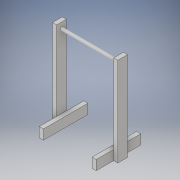
# Autodesk Inventor part: Perch
Saved by Autodesk Inventor 2017 (Build 210142000, 142)
## iProperties
Created: 2017-04-14
Part Number: Perch
Material: Generic
Document SubType Name: Modeling
Designer: Alex Tacescu
Density: 1 g/cm^3
Appearance: Default
Author: Alex Tacescu
Autodesk Inventor part; units mm, degrees
ref_plane "YZ Plane" through (0, 0, 0) normal (1, 0, 0) x (0, 1, 0)
ref_plane "XZ Plane" through (0, 0, 0) normal (0, 1, 0) x (-1, 0, 0)
ref_plane "XY Plane" through (0, 0, 0) normal (0, 0, 1) x (1, 0, 0)
sketch "Sketch1" plane through (0, 0, 0) normal (0, 1, 0) x (-1, 0, 0)
  line L0 (0, -284.48) -> (0, 284.48) projected
  line L1 (-364.49, 0) -> (364.49, 0) projected
  line L2 (260.35, 203.2) -> (222.25, 203.2)
  line L3 (222.25, 203.2) -> (222.25, -203.2)
  line L4 (222.25, -203.2) -> (260.35, -203.2)
  line L5 (260.35, -203.2) -> (260.35, 203.2)
  line L6 (260.35, 203.2) -> (222.25, -203.2) construction
  line L7 (222.25, 203.2) -> (260.35, -203.2) construction
  line L8 (-260.35, 203.2) -> (-222.25, 203.2)
  line L9 (-222.25, 203.2) -> (-222.25, -203.2)
  line L10 (-222.25, -203.2) -> (-260.35, -203.2)
  line L11 (-260.35, -203.2) -> (-260.35, 203.2)
  line L12 (-260.35, 203.2) -> (-222.25, -203.2) construction
  line L13 (-222.25, 203.2) -> (-260.35, -203.2) construction
  point P0 (0, 0)
  point P1 (241.3, 0)
  point P2 (-241.3, 0)
  dimension "d0" = 38.1
  dimension "d1" = 406.4
  dimension "d3" = 260.35
  constraints: 24 end point, 5 symmetric about line, 4 midpoint, 2 parallel, 1 horizontal, 1 perpendicular, 1 point on line
  measures "d0" distance of L3.end L4.end
  measures "d1" distance of L4.end L2.start
  measures "d3" distance between parallel lines of L0 L5
extrude "Extrusion1" add sketch "Sketch1" along normal blind 88.9
sketch "Sketch2" plane through (0, 0, 0) normal (0, -1, 0) x (1, 0, 0)
  line L0 (-260.35, 203.2) -> (-222.25, 203.2) projected
  line L1 (-260.35, -203.2) -> (-260.35, 203.2) projected
  line L2 (-222.25, -203.2) -> (-260.35, -203.2) projected
  line L3 (-222.25, 203.2) -> (-222.25, -203.2) projected
  line L4 (260.35, 203.2) -> (222.25, 203.2) projected
  line L5 (222.25, 203.2) -> (222.25, -203.2) projected
  line L6 (222.25, -203.2) -> (260.35, -203.2) projected
  line L7 (260.35, -203.2) -> (260.35, 203.2) projected
  line L8 (-417.83, 0) -> (417.83, 0) projected
  line L9 (-298.45, -44.45) -> (-260.35, -44.45)
  line L10 (-260.35, -44.45) -> (-260.35, 44.45)
  line L11 (-260.35, 44.45) -> (-298.45, 44.45)
  line L12 (-298.45, 44.45) -> (-298.45, -44.45)
  line L13 (-298.45, -44.45) -> (-260.35, 44.45) construction
  line L14 (-260.35, -44.45) -> (-298.45, 44.45) construction
  line L15 (0, 284.48) -> (0, -284.48) projected
  line L16 (298.45, -44.45) -> (260.35, -44.45)
  line L17 (260.35, -44.45) -> (260.35, 44.45)
  line L18 (260.35, 44.45) -> (298.45, 44.45)
  line L19 (298.45, 44.45) -> (298.45, -44.45)
  line L20 (298.45, -44.45) -> (260.35, 44.45) construction
  line L21 (260.35, -44.45) -> (298.45, 44.45) construction
  point P0 (0, 0)
  point P1 (-279.4, 0)
  point P2 (279.4, 0)
  dimension "d6" = 38.1
  dimension "d7" = 88.9
  constraints: 24 end point, 5 symmetric about line, 4 midpoint, 2 parallel, 2 point on line, 1 horizontal, 1 perpendicular
  measures "d6" distance of L10.end L11.end
  measures "d7" distance of L11.end L9.start
extrude "Extrusion2" add sketch "Sketch2" against normal blind 812.8 contours L1 L8 L12 L11 | L1 L9 L12 L8 | L18 L19 L8 L7 | L8 L19 L16 L7
sketch "Sketch3" plane through (298.45, 0, 44.45) normal (1, 0, 0) x (0, 0, -1)
  line L0 (88.9, 0) -> (0, 0) projected
  line L1 (88.9, 0) -> (88.9, 812.8) projected
  line L2 (0, 812.8) -> (88.9, 812.8) projected
  line L3 (0, 0) -> (0, 812.8) projected
  line L4 (44.45, -162.56) -> (44.45, 975.36) projected
  circle A0 centre (44.45, 762) radius 12.7
  point P0 (44.45, 0)
  dimension "d10" = 25.4
  dimension "d11" = 762
  constraints: 1 centre point, 1 point on line
  measures "d10" diameter of A0
  measures "d11" distance from line of L0 A0.centre
extrude "Extrusion3" add sketch "Sketch3" against normal up to surface (596.9 mm away) contours A0 L4 | L4 A0
body "Solid1"
